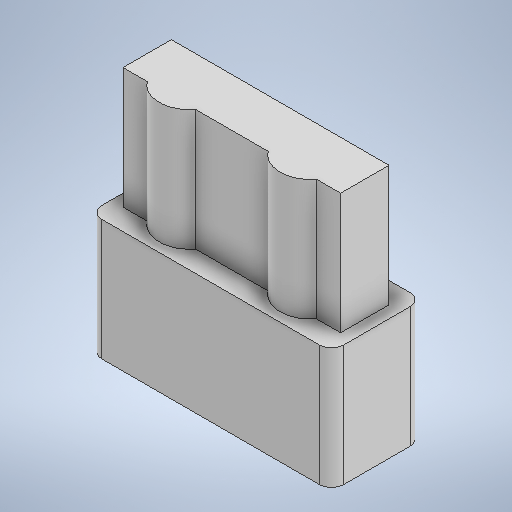
# Autodesk Inventor part: zaslepka
Saved by Autodesk Inventor 2025.2 (Build 292293000, 293)
## iProperties
Created: 2025-11-26
Part Number: zaslepka
Material: Ogólny
Document SubType Name: Modeling
Designer: juras
Density: 1 g/cm^3
Appearance: Domyślna
Author: juras
Autodesk Inventor part; units mm, degrees
ref_plane "YZ Plane" through (0, 0, 0) normal (1, 0, 0) x (0, 1, 0)
ref_plane "XZ Plane" through (0, 0, 0) normal (0, 1, 0) x (-1, 0, 0)
ref_plane "XY Plane" through (0, 0, 0) normal (0, 0, 1) x (1, 0, 0)
sketch "Szkic2" plane through (0, 0, 0) normal (0, 1, 0) x (-1, 0, 0)
  line L0 (-20, -7.5) -> (20, -7.5)
  line L1 (20, -7.5) -> (20, 7.5)
  line L2 (20, 7.5) -> (-20, 7.5)
  line L3 (-20, 7.5) -> (-20, -7.5)
  line L4 (-20, -7.5) -> (20, 7.5) construction
  line L5 (20, -7.5) -> (-20, 7.5) construction
  point P0 (0, 0)
  dimension "d12" = 40
  dimension "d13" = 15
  constraints: 12 end point, 2 midpoint, 2 parallel, 1 horizontal, 1 perpendicular
  measures "d12" distance of L2.end L1.end
  measures "d13" distance of L1.end L0.end
extrude "Wyciągnięcie proste1" add sketch "Szkic2" along normal mid plane 20
sketch "Szkic3" plane through (0, 10, 0) normal (0, 1, 0) x (1, 0, 0)
  line L0 (18, 4) -> (-18, 4)
  line L1 (-18, 4) -> (-18, -4)
  line L2 (-18, -4) -> (18, -4)
  line L3 (18, -4) -> (18, 4)
  line L4 (18, 4) -> (-18, -4) construction
  line L5 (-18, 4) -> (18, -4) construction
  circle A0 centre (10, -1) radius 5
  circle A1 centre (-10, -1) radius 5
  circle A2 centre (10, -1) radius 2.5
  circle A3 centre (-10, -1) radius 2.5
  point P0 (0, 0)
  point P1 (6, -4)
  point P2 (10, 4)
  point P3 (-10, 4)
  point P4 (-6, -4)
  point P5 (14, -4)
  point P6 (-14, -4)
  dimension "d16" = 36
  dimension "d17" = 8
  dimension "d18" = 10
  dimension "d19" = 8
  dimension "d20" = 5
  dimension "d21" = 10
  dimension "d22" = 5
  dimension "d23" = 8
  dimension "d24" = 5
  dimension "d25" = 5
  constraints: 12 end point, 4 centre point, 2 coincident, 2 midpoint, 2 parallel, 1 horizontal, 1 perpendicular
  measures "d16" distance of L2.end L1.end
  measures "d17" distance of L1.end L0.end
  measures "d18" diameter of A0
  measures "d19" distance from line of A0.centre L3
  measures "d20" distance from line of L0 A0.centre
  measures "d21" diameter of A1
  measures "d22" distance from line of L0 A1.centre
  measures "d23" distance from line of L1 A1.centre
  measures "d24" diameter of A2
  measures "d25" diameter of A3
extrude "Wyciągnięcie proste2" add sketch "Szkic3" along normal blind 20 contours L3 L2 A0 L0 | A0 L2 A1 L0 | A0 L2 | A1 L2 L1 L0 | A1 L2 | L2 A0 | L2 A1 | A2 | A3
fillet "Zaokrąglenie1" radius 2 4 edges at (20, 0, 7.5) (-20, 0, 7.5) (20, 0, -7.5) (-20, 0, -7.5)
